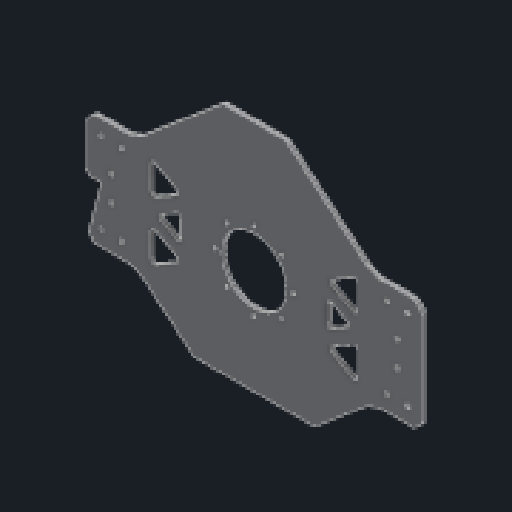
# Autodesk Inventor part: Root
Saved by Autodesk Inventor 2025.2 (Build 292293000, 293)
## iProperties
Created: 2020-05-07
Part Number: Root
Material: Generic
Document SubType Name: Sheet Metal
Designer: valer
Density: 1 g/cm^3
Sheet Metal Rule: Default
Appearance: Default
Author: valer
Autodesk Inventor part; units mm, degrees
ref_plane "YZ Plane" through (0, 0, 0) normal (1, 0, 0) x (0, 1, 0)
ref_plane "XZ Plane" through (0, 0, 0) normal (0, 1, 0) x (-1, 0, 0)
ref_plane "XY Plane" through (0, 0, 0) normal (0, 0, 1) x (1, 0, 0)
sketch "Base" plane through (0, 0, 0) normal (0, 0, 1) x (1, 0, 0)
  circle A0 centre (-56.25, 0) radius 2.75 construction
  circle A1 centre (0, -56.25) radius 2.75 construction
  circle A2 centre (0, 56.25) radius 2.75 construction
  circle A3 centre (39.7748, -39.7748) radius 2.75 construction
  circle A4 centre (-39.7748, 39.7748) radius 2.75 construction
  circle A5 centre (-39.7748, -39.7748) radius 2.75 construction
  circle A6 centre (39.7748, 39.7748) radius 2.75 construction
  circle A7 centre (56.25, 0) radius 2.75 construction
  circle A8 centre (0, 0) radius 45 construction
  circle A9 centre (0, 0) radius 61
  line L0 (260, 80) -> (-260, 80) construction
  line L1 (0, -210) -> (0, 210) construction
  line L2 (-364, 0) -> (364, 0) construction
  line L3 (-260, 80) -> (-190, 80)
  line L4 (-190, 80) -> (-190, 0)
  line L5 (-190, 0) -> (-260, 0)
  line L6 (-260, 0) -> (-260, 80)
  line L7 (86.6025, -150) -> (-86.6025, -150)
  line L8 (-86.6025, -150) -> (-173.2051, 0)
  line L9 (-173.2051, 0) -> (-86.6025, 150)
  line L10 (-86.6025, 150) -> (86.6025, 150)
  line L11 (86.6025, 150) -> (173.2051, 0)
  line L12 (173.2051, 0) -> (86.6025, -150)
  line L13 (-190, 0) -> (-86.6025, 150) construction
  line L14 (260, 80) -> (190, 80)
  line L15 (190, 80) -> (190, 0)
  line L16 (190, 0) -> (260, 0)
  line L17 (260, 0) -> (260, 80)
  line L18 (190, 0) -> (86.6025, 150) construction
  line L19 (-260, -80) -> (-190, -80)
  line L20 (-190, -80) -> (-190, 0)
  line L21 (-190, 0) -> (-260, 0)
  line L22 (-260, 0) -> (-260, -80)
  line L23 (-190, 0) -> (-86.6025, -150) construction
  line L24 (260, 0) -> (260, -80)
  line L25 (260, -80) -> (190, -80)
  line L26 (190, -80) -> (190, 0)
  line L27 (190, 0) -> (260, 0)
  line L28 (190, 0) -> (86.6025, -150) construction
  circle A10 centre (0, 0) radius 46.5
  circle A11 centre (-56.25, 0) radius 2.25
  circle A12 centre (-39.7748, -39.7748) radius 2.25
  circle A13 centre (0, -56.25) radius 2.25
  circle A14 centre (39.7748, -39.7748) radius 2.25
  circle A15 centre (56.25, 0) radius 2.25
  circle A16 centre (39.7748, 39.7748) radius 2.25
  circle A17 centre (0, 56.25) radius 2.25
  circle A18 centre (-39.7748, 39.7748) radius 2.25
  line L29 (-190, 80) -> (-86.6025, 150)
  line L30 (86.6025, 150) -> (190, 80)
  line L31 (-190, -80) -> (-86.6025, -150)
  line L32 (86.6025, -150) -> (190, -80)
  point P0 (0, 0)
  point P1 (210, 0)
  point P2 (170, 5.5514)
  point P3 (170, -5.5514)
  point P4 (173.2051, 0)
  point P5 (173.2051, 0)
  point P6 (-170, 5.5514)
  point P7 (-173.2051, 0)
  point P8 (-173.2051, 0)
  point P9 (-170, -5.5514)
  point P10 (173.2051, 0)
  point P11 (190, 0)
  point P12 (190, 0)
  point P13 (-190, 0)
  point P14 (-173.2051, 0)
  point P15 (-190, 0)
  point P16 (-173.2051, 0)
  dimension "d89" = 80
  dimension "d90" = 70
  dimension "d91" = 1.5
  dimension "d92" = 4.5
  dimension "d157" = 150
  dimension "d162" = 380
  measures "d89" distance between parallel lines of L0 L5
  measures "d90" distance between parallel lines of L4 L6
  measures "d91" radial gap between concentric circles of A10 A8
  measures "d92" diameter of A11
  measures "d157" distance from line of L7 A8.centre
  measures "d162" distance between parallel lines of L20 L26
extrude "Plate1" add sketch "Base" against normal blind 5 contours A9 | L3 L4 L5 L6 | L29 L9 L8 L31 L20 L4 | L5 L20 L19 L22 | L10 L11 L12 L7 L8 L9 | L30 L15 L26 L32 L12 L11 | L14 L17 L16 L15 | L16 L24 L25 L26
sketch "LegMountHoles" plane through (0, 0, -5) normal (0, 0, -1) x (-1, 0, 0)
  line L0 (-308.1685, 0) -> (-220, 0) construction
  line L1 (-260, 80) -> (-190, 80) construction
  line L2 (-225, 80) -> (-225, 0) construction
  line L3 (-210, 58) -> (-240, 58) construction
  circle A0 centre (-210, 58) radius 3
  circle A1 centre (-240, 58) radius 3
  circle A2 centre (-225, 18) radius 3
  line L4 (369.348, 0) -> (-396.0879, 0) construction
  line L5 (0, -210) -> (0, 210) construction
  circle A3 centre (210, 58) radius 3
  circle A4 centre (240, 58) radius 3
  circle A5 centre (225, 18) radius 3
  circle A6 centre (-210, -58) radius 3
  circle A7 centre (-240, -58) radius 3
  circle A8 centre (-225, -18) radius 3
  circle A9 centre (210, -58) radius 3
  circle A10 centre (240, -58) radius 3
  circle A11 centre (225, -18) radius 3
  line L6 (-190, 80) -> (-86.6025, 150) projected
  line L7 (-260, -80) -> (-260, 80) projected
  point P0 (0, 0)
  point P1 (-225, 58)
  dimension "d93" = 6
  dimension "d94" = 30
  dimension "d95" = 40
  dimension "d161" = 18
  constraints: 12 centre point, 9 symmetric about line, 6 end point, 4 point on line, 3 horizontal, 2 coincident, 2 equal radius, 2 midpoint, 1 collinear, 1 perpendicular, 10 other
  measures "d93" diameter of A0
  measures "d94" distance of L3.start L3.end
  measures "d95" distance from line of L3 A2.centre
  measures "d161" distance from line of L4 A2.centre
extrude "LegMountHolesFeature" cut sketch "LegMountHoles" against normal blind 5
chamfer "OutsideChamfersFeature" distance 10 angle 45 8 edges at (-260, -80, -2.5) (-190, -80, -2.5) (190, -80, -2.5) (260, -80, -2.5) (-260, 80, -2.5) (-190, 80, -2.5) (190, 80, -2.5) (260, 80, -2.5)
fillet "OutsideFilletsFeature" radius 8 17 edges at (200, 80, -2.5) (250, 80, -2.5) (260, 70, -2.5) (250, -80, -2.5) (200, -80, -2.5) (86.6025, -150, -2.5) (-86.6025, -150, -2.5) (-200, -80, -2.5) (-250, -80, -2.5) (-260, -70, -2.5) (-260, 70, -2.5) (-250, 80, -2.5) (-200, 80, -2.5) (-181.7192, 85.6061, -2.5) (181.7192, 85.6061, -2.5) (181.7192, -85.6061, -2.5) (-181.7192, -85.6061, -2.5)
sketch "TrianglePattern" plane through (0, 0, -5) normal (0, 0, -1) x (-1, 0, 0)
  line L0 (-148.3013, -66.7074) -> (-105, -41.7074)
  line L1 (-105, -41.7074) -> (-148.3013, -16.7074)
  line L2 (-148.3013, -16.7074) -> (-148.3013, -66.7074)
  line L3 (-139.641, 0) -> (-105, -20)
  line L4 (-105, -20) -> (-105, 20)
  line L5 (-105, 20) -> (-139.641, 0)
  line L6 (364, 0) -> (-364, 0) construction
  line L7 (-148.3013, 66.7074) -> (-105, 41.7074)
  line L8 (-105, 41.7074) -> (-148.3013, 16.7074)
  line L9 (-148.3013, 16.7074) -> (-148.3013, 66.7074)
  line L10 (0, -210) -> (0, 210) construction
  line L11 (148.3013, -66.7074) -> (105, -41.7074)
  line L12 (105, -41.7074) -> (148.3013, -16.7074)
  line L13 (148.3013, -16.7074) -> (148.3013, -66.7074)
  line L14 (139.641, 0) -> (105, -20)
  line L15 (105, -20) -> (105, 20)
  line L16 (105, 20) -> (139.641, 0)
  line L17 (148.3013, 16.7074) -> (148.3013, 66.7074)
  line L18 (148.3013, 66.7074) -> (105, 41.7074)
  line L19 (105, 41.7074) -> (148.3013, 16.7074)
  line L20 (-105, 41.7074) -> (-105, 20) construction
  line L21 (-105, 41.7074) -> (-148.3013, 41.7074) construction
  line L22 (-105, -41.7074) -> (-148.3013, -41.7074) construction
  point P0 (0, 0)
  dimension "d149" = 30
  dimension "d150" = 18.7992
  dimension "d151" = 30
  dimension "d152" = 30
  dimension "d153" = 18.7992
  dimension "d154" = 40
  dimension "d155" = 50
  dimension "d156" = 105
  constraints: 42 end point, 12 symmetric about line, 4 parallel, 2 midpoint, 1 collinear, 1 perpendicular, 1 point on line
  measures "d149" angle of L6 L5
  measures "d150" distance between parallel lines of L5 L8
  measures "d151" angle of L8 L21
  measures "d152" angle of L22 L1
  measures "d153" distance between parallel lines of L1 L3
  measures "d154" distance of L3.end L4.end
  measures "d155" distance of L9.start L9.end
  measures "d156" distance from line of L4 point (0, 0)
extrude "TriangleHolesFeature" cut sketch "TrianglePattern" against normal blind 5
fillet "TriangleHoleFilletsFeature" radius 4 16 edges at (105, -20, -2.5) (105, 20, -2.5) (139.641, 0, -2.5) (105, -41.7074, -2.5) (148.3013, -16.7074, -2.5) (148.3013, -66.7074, -2.5) (105, 41.7074, -2.5) (148.3013, 66.7074, -2.5) (148.3013, 16.7074, -2.5) (-148.3013, 16.7074, -2.5) (-105, 41.7074, -2.5) (-139.641, 0, -2.5) (-105, 20, -2.5) (-105, -20, -2.5) (-148.3013, -16.7074, -2.5) (-105, -41.7074, -2.5)
equation "\"d97\" = Thickness"
equation "\"d33\" = Thickness"
equation "\"BendRadius\" = Thickness"
equation "\"BendReliefWidth\" = Thickness"
equation "\"BendReliefDepth\" = 0.5 * Thickness"
equation "\"TransitionRadius\" = BendRadius"
equation "\"JacobiRadiusSize\" = BendRadius"
equation "\"GapSize\" = Thickness"
equation "\"Thickness\" = 5"
body "Solid1"
